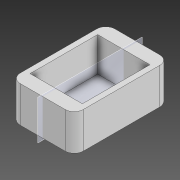
# Autodesk Inventor part: CH_01_0038_kradex_place_holder
Saved by Autodesk Inventor 2022 (Build 260153000, 153)
## iProperties
Created: 2022-05-09
Part Number: CH_01_0038_kradex_place_holder
Material: Generic
Document SubType Name: Modeling
Designer: Tomasz Krakowski
Density: 1 g/cm^3
Appearance: Default
Author: Tomasz Krakowski
Autodesk Inventor part; units mm, degrees
ref_plane "XZ Plane" through (0, 0, 0) normal (0, 1, 0) x (-1, 0, 0)
ref_plane "XY Plane" through (0, 0, 0) normal (0, 0, 1) x (1, 0, 0)
sketch "Sketch1" plane through (0, 0, 0) normal (0, 1, 0) x (-1, 0, 0)
  line L0 (-35, 52.5) -> (35, 52.5)
  line L1 (35, 52.5) -> (35, -52.5)
  line L2 (35, -52.5) -> (-35, -52.5)
  line L3 (-35, -52.5) -> (-35, 52.5)
  line L4 (-35, 52.5) -> (35, -52.5) construction
  line L5 (35, 52.5) -> (-35, -52.5) construction
  point P0 (0, 0)
  dimension "d0" = 105
  dimension "d1" = 70
  constraints: 12 end point, 2 midpoint, 2 parallel, 1 horizontal, 1 perpendicular
  measures "d0" distance of L0.end L1.end
  measures "d1" distance between parallel lines of L3 L1
extrude "Extrusion1" add sketch "Sketch1" along normal blind 40
fillet "Fillet1" radius 10 4 edges at (-35, 20, 52.5) (35, 20, 52.5) (-35, 20, -52.5) (35, 20, -52.5)
sketch "Sketch2" plane through (0, 40, 0) normal (0, 1, 0) x (1, 0, 0)
  line L0 (29, -37.5) -> (-29, -37.5)
  line L1 (-29, -37.5) -> (-29, 37.5)
  line L2 (-29, 37.5) -> (29, 37.5)
  line L3 (29, 37.5) -> (29, -37.5)
  line L4 (29, -37.5) -> (-29, 37.5) construction
  line L5 (-29, -37.5) -> (29, 37.5) construction
  point P0 (0, 0)
  dimension "d5" = 58
  dimension "d6" = 75
  constraints: 12 end point, 2 midpoint, 2 parallel, 1 horizontal, 1 perpendicular
  measures "d5" distance between parallel lines of L3 L1
  measures "d6" distance between parallel lines of L2 L0
extrude "Extrusion2" cut sketch "Sketch2" against normal blind 38
body "Solid1"
